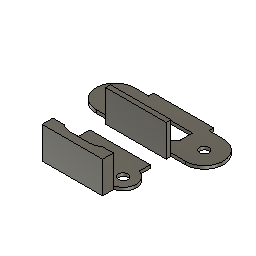
Cutting Templates v1 (Autodesk Fusion 360 design; units mm, degrees)
Autodesk Fusion 360 part; units mm, degrees
sketch "Sketch1" plane through (0, 0, 0) normal (0, 0, 1) x (1, 0, 0)
  line L0 (-14, 0) -> (14, 0) construction
  line L1 (-14, -6) -> (14, -6)
  arc A0 (14, -6) -> (14, 6) centre (14, 0) ccw
  line L2 (14, 6) -> (-14, 6)
  arc A1 (-14, 6) -> (-14, -6) centre (-14, 0) ccw
  line L3 (-14, 0) -> (14, 0) construction
  line L4 (-7.5, 2.75) -> (7.5, 2.75)
  line L5 (7.5, 2.75) -> (7.5, -1.15)
  line L6 (7.5, -1.15) -> (5.9, -2.75)
  line L7 (5.9, -2.75) -> (-5.9, -2.75)
  line L8 (-5.9, -2.75) -> (-7.5, -1.15)
  line L9 (-7.5, -1.15) -> (-7.5, 2.75)
  circle A2 centre (-14, 0) radius 1.5
  circle A3 centre (14, 0) radius 1.5
  line L10 (-9.5, 7.5) -> (9.5, 7.5)
  line L11 (9.5, 7.5) -> (9.5, -7.5)
  line L12 (9.5, -7.5) -> (-9.5, -7.5)
  line L13 (-9.5, -7.5) -> (-9.5, 7.5)
  point P0 (0, 2.75)
  dimension "d1" = 28
  dimension "d2" = 6
  dimension "d3" = 15
  dimension "d4" = 5.5
  dimension "d5" = 3.9
  dimension "d6" = 2.75
  dimension "d7" = 3
  dimension "d8" = 3
  dimension "d21" = 15
  dimension "d22" = 7.5
  dimension "d23" = 19
  dimension "d24" = 9.5
  constraint horizontal L0
  constraint midpoint origin L0
  constraint tangent L1 A0
  constraint tangent A0 L2
  constraint parallel L1 L2
  constraint tangent L2 A1
  constraint tangent L1 A1
  constraint coincident L0.end A0.centre
  constraint parallel L0 L3
  constraint coincident L0.start A1.centre
  constraint horizontal L4
  constraint perpendicular L0 L5
  constraint perpendicular L5 L7
  constraint perpendicular L6 L8
  constraint vertical L9
  constraint coincident L4 P0
  constraint midpoint L4 P0
  constraint vertical origin P0
  constraint equal L5 L9
  constraint equal L6 L8
  constraint concentric A1 A2
  constraint concentric A0 A3
  constraint horizontal L10
  constraint vertical L11
  constraint horizontal L12
  constraint vertical L13
  measures "d1" distance of L0.start L0.end
  measures "d2" radius of A0
  measures "d3" distance of L4.start L4.end
  measures "d4" distance of L4 L7
  measures "d5" distance of L4.end L5.end
  measures "d6" distance of L3 L7
  measures "d7" diameter of A3
  measures "d8" diameter of A2
  measures "d21" distance of L10.end L11.end
  measures "d22" distance of origin L10
  measures "d23" distance of L10.start L10.end
  measures "d24" distance of origin L11
extrude "Extrude1" add sketch "Sketch1" along normal blind 1 contours L1 L2 A1 L13 | L1 L2 L11 L13 | L1 A0 L2 L11 | L2 L10 L11 L13 makes body 1
extrude "Extrude3" add sketch "Sketch1" along normal blind 10 contours L1 L11 L12 L13 bodies 1
sketch "Sketch2" plane through (0, 0, 0) normal (0, 0, 1) x (1, 0, 0)
  line L0 (-8.5, -24.1) -> (8.5, -24.1)
  arc A0 (8.5, -24.1) -> (8.5, -15.9) centre (8.5, -20) ccw
  line L1 (8.5, -15.9) -> (-8.5, -15.9)
  arc A1 (-8.5, -15.9) -> (-8.5, -24.1) centre (-8.5, -20) ccw
  line L2 (-8.5, -20) -> (8.5, -20) construction
  line L3 (-2.875, -21.625) -> (2.875, -21.625)
  arc A2 (2.875, -21.625) -> (2.875, -18.375) centre (2.875, -20) ccw
  line L4 (2.875, -18.375) -> (-2.875, -18.375)
  arc A3 (-2.875, -18.375) -> (-2.875, -21.625) centre (-2.875, -20) ccw
  line L5 (-2.875, -20) -> (2.875, -20) construction
  line L6 (4.5, -17.2515) -> (4.5, -22.6673) construction
  line L7 (-2.875, -25.15) -> (2.875, -25.15)
  arc A4 (2.875, -25.15) -> (2.875, -14.85) centre (2.875, -20) ccw
  line L8 (2.875, -14.85) -> (-2.875, -14.85)
  arc A5 (-2.875, -14.85) -> (-2.875, -25.15) centre (-2.875, -20) ccw
  line L9 (-2.875, -20) -> (2.875, -20) construction
  circle A6 centre (8.5, -20) radius 1.5
  circle A7 centre (-8.5, -20) radius 1.5
  line L10 (-9.5, -12.5) -> (9.5, -12.5)
  line L11 (9.5, -12.5) -> (9.5, -27.5)
  line L12 (9.5, -27.5) -> (-9.5, -27.5)
  line L13 (-9.5, -27.5) -> (-9.5, -12.5)
  point P0 (0, -20)
  point P1 (0, -20)
  dimension "d11" = 17
  dimension "d12" = 4.1
  dimension "d13" = 20
  dimension "d14" = 3.25
  dimension "d15" = 4.5
  dimension "d16" = 10.3
  dimension "d17" = 3
  dimension "d18" = 3
  dimension "d25" = 19
  dimension "d26" = 9.5
  dimension "d27" = 15
  dimension "d28" = 7.5
  constraint tangent L0 A0
  constraint tangent A0 L1
  constraint parallel L0 L1
  constraint tangent L1 A1
  constraint tangent L0 A1
  constraint horizontal L2
  constraint coincident L2 P1
  constraint midpoint L2 P1
  constraint vertical origin P1
  constraint tangent L3 A2
  constraint tangent A2 L4
  constraint parallel L3 L4
  constraint tangent L4 A3
  constraint tangent L3 A3
  constraint coincident L2 A2.centre
  constraint parallel L2 L5
  constraint vertical L6
  constraint midpoint P1 L5
  constraint tangent A2 L6
  constraint tangent L7 A4
  constraint tangent A4 L8
  constraint parallel L7 L8
  constraint tangent L8 A5
  constraint tangent L7 A5
  constraint parallel L2 L9
  constraint coincident P1 P0
  constraint midpoint L9 P1
  constraint coincident A2.centre L5.end
  constraint concentric A0 A6
  constraint concentric A1 A7
  constraint horizontal L10
  constraint vertical L11
  constraint horizontal L12
  constraint vertical L13
  measures "d11" distance of A1.centre A0.centre
  measures "d12" radius of A0
  measures "d13" distance of origin P1
  measures "d14" distance of L3 L4
  measures "d15" distance of P1 L6
  measures "d16" distance of L7 L8
  measures "d17" diameter of A7
  measures "d18" diameter of A6
  measures "d25" distance of L11.end L12.end
  measures "d26" distance of P1 L11
  measures "d27" distance of L10.end L11.end
  measures "d28" distance of L2 L10
extrude "Extrude2" add sketch "Sketch2" along normal blind 1 separate body contours L0 A1 A5 A7 L13 | L0 L1 A4 A5 A6 A7 | L0 L7 A4 A5 | A1 A7 L13 | L0 A0 A4 A6 L11 | A0 L1 A1 A4 L8 A5 L10 L11 L13 | L1 A1 A5 A7 L13 | A0 A6 L11 | A0 L1 A4 A6 L11 | L1 A4 L8 A5 makes body 2
extrude "Extrude4" add sketch "Sketch2" along normal up to surface (10 mm away) contours L0 A0 A1 L7 A4 A5 L11 L12 L13 bodies 2
equation "d6 = d4 / 2"
equation "d22 = d21 / 2"
equation "d24 = d23 / 2"
equation "d26 = d25 / 2"
equation "d28 = d27 / 2"
named bodies: "HDMI", "USBC"
